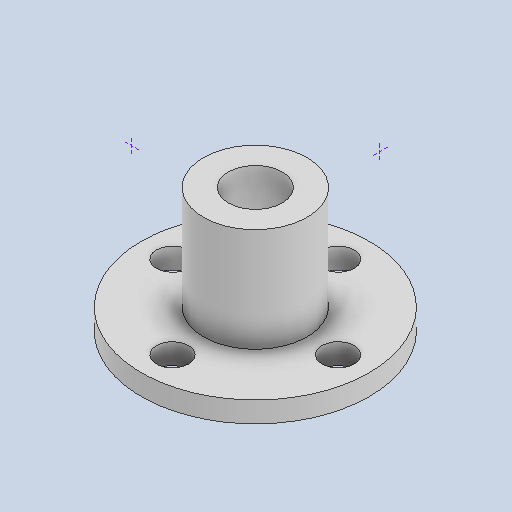
# Autodesk Inventor part: Муфта
Saved by Autodesk Inventor 2024.2 (Build 282272000, 272)
## iProperties
Created: 2025-11-19
Part Number: Муфта
Material: Типовые
Document SubType Name: Modeling
Designer: Zakhar
Density: 1 g/cm^3
Appearance: По умолчанию
Mass: 1.11751 g
Surface Area: 12.9653 cm^2
Volume: 1.11751 cm^3
Author: Zakhar
Autodesk Inventor part; units mm, degrees
ref_plane "YZ Plane" through (0, 0, 0) normal (1, 0, 0) x (0, 1, 0)
ref_plane "XZ Plane" through (0, 0, 0) normal (0, 1, 0) x (-1, 0, 0)
sketch "Эскиз1" plane through (0, 0, 0) normal (0, 1, 0) x (-1, 0, 0)
  circle A0 centre (0, 0) radius 5
  circle A1 centre (0, 0) radius 2.6
  circle A2 centre (0, 0) radius 11
  circle A3 centre (8, 0) radius 1.55
  circle A4 centre (-8, 0) radius 1.55
  circle A5 centre (0, 8) radius 1.55
  circle A6 centre (0, -8) radius 1.55
  dimension "d0" = 5.2
  dimension "d1" = 10
  dimension "d2" = 22
  dimension "d3" = 3.1
  dimension "d4" = 3.1
  dimension "d5" = 16
  dimension "d6" = 8
  dimension "d7" = 3.1
  dimension "d8" = 3.1
  dimension "d9" = 8
  dimension "d10" = 8
  dimension "d11" = 16
  constraints: 7 centre point, 3 coincident, 1 other
  measures "d0" diameter of A1
  measures "d1" diameter of A0
  measures "d2" diameter of A2
  measures "d3" diameter of A4
  measures "d4" diameter of A3
  measures "d5" distance of A4.centre A3.centre
  measures "d6" distance of A2.centre A4.centre
  measures "d7" diameter of A5
  measures "d8" diameter of A6
  measures "d9" distance of point (0, 0) A6.centre
  measures "d10" distance of point (0, 0) A5.centre
  measures "d11" distance of A6.centre A5.centre
extrude "Выдавливание1" add sketch "Эскиз1" along normal blind 2 contours A2
extrude "Выдавливание2" add sketch "Эскиз1" along normal blind 12 contours A0
sketch "Эскиз2" plane through (0, 0, 0) normal (1, 0, 0) x (0, 1, 0)
  point P0 (0, 0)
  point P1 (-0.4556, -12.0524)
  point P2 (8.9773, -12.0404)
sketch "Эскиз3" plane through (0, 0, 0) normal (0, 0, 1) x (1, 0, 0)
  point P0 (0, 0)
  point P1 (-11.9191, -0.1213)
  point P2 (-11.9191, 9.5232)
ref_plane "РабПлоскость1" through (0, -0.4556, -12.0524) normal (0.711, -0.0009, 0.7032) x (0, 1, 0.0013)
sketch "Эскиз4" plane through (0, -0.4556, -12.0524) normal (0.711, -0.0009, 0.7032) x (0, 1, 0.0013)
  circle A0 centre (6.1565, 8.569) radius 1.5
  point P0 (0.4709, 8.569)
  dimension "d16" = 3
  constraints: 1 centre point
  measures "d16" diameter of A0
extrude "Выдавливание3" cut sketch "Эскиз4" along normal up to surface
